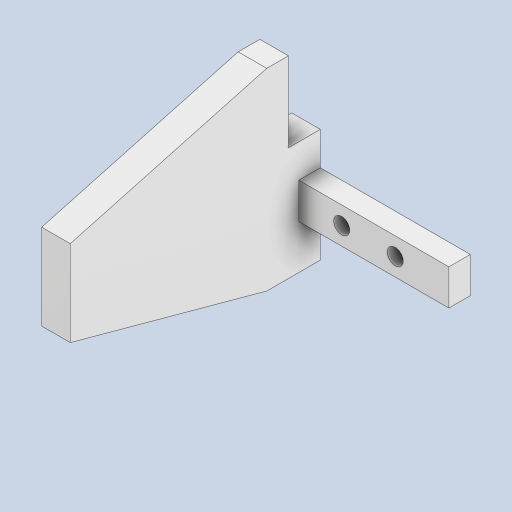
# Autodesk Inventor part: right-nail
Saved by Autodesk Inventor 2023 (Build 270158000, 158)
## iProperties
Created: 2024-11-28
Part Number: right-nail
Material: ABS プラスチック
Document SubType Name: Modeling
Designer: kiyo
Density: 1.06 g/cm^3
Appearance: 滑らか - 白
Author: kiyo
Autodesk Inventor part; units mm, degrees
ref_plane "YZ Plane" through (0, 0, 0) normal (1, 0, 0) x (0, 1, 0)
ref_plane "XZ Plane" through (0, 0, 0) normal (0, 1, 0) x (-1, 0, 0)
ref_plane "XY Plane" through (0, 0, 0) normal (0, 0, 1) x (1, 0, 0)
sketch "スケッチ2" plane through (0, 0, 0) normal (1, 0, 0) x (0, 1, 0)
  line L0 (-50, 41.625) -> (0, 41.625)
  line L1 (0, 41.625) -> (0, 31.625)
  line L2 (0, 31.625) -> (-50, 31.625)
  line L3 (-50, 31.625) -> (-50, 41.625)
  line L4 (0, 31.625) -> (-8, 31.625)
  line L5 (-8, 31.625) -> (-8, 0)
  line L6 (-8, 0) -> (0, 0)
  line L7 (0, 0) -> (0, 31.625)
  circle A0 centre (-20, 36.625) radius 2.25
  circle A1 centre (-35, 36.625) radius 2.25
  line L8 (-8, 31.625) -> (0, 31.625)
  line L9 (0, 31.625) -> (0, 54)
  line L10 (0, 54) -> (-8, 54)
  line L11 (-8, 54) -> (-8, 31.625)
  point P0 (-8, 31.625)
  point P1 (-8, 41.625)
  point P2 (0, 41.625)
  dimension "d7" = 50
  dimension "d8" = 10
  dimension "d10" = 8
  dimension "d11" = 4.5
  dimension "d12" = 4.5
  dimension "d13" = 15
  dimension "d14" = 20
  dimension "d15" = 5
  dimension "d16" = 5
  dimension "d27" = 54
  dimension "d28" = 12.375
  constraints: 24 end point, 6 parallel, 3 horizontal, 3 perpendicular, 2 centre point, 1 coincident, 1 collinear
  measures "d7" distance of L0.start L0.end
  measures "d8" distance between parallel lines of L2 L0
  measures "d10" distance of L5.end L6.end
  measures "d11" diameter of A0
  measures "d12" diameter of A1
  measures "d13" distance of A0.centre A1.centre
  measures "d14" distance from line of L1 A0.centre
  measures "d15" distance from line of L0 A0.centre
  measures "d16" distance from line of L0 A1.centre
  measures "d27" distance between parallel lines of L6 L10
  measures "d28" distance between parallel lines of L0 L10
extrude "押し出し2" add sketch "スケッチ2" along normal blind 6 contours L0 L11 L2 L3
extrude "押し出し5" add sketch "スケッチ2" along normal blind 70 contours L11 L10 L9 L0 | L0 L1 L2 L11 | L2 L7 L6 L5
sketch "スケッチ4" plane through (0, 0, 54) normal (0, 1, 0) x (1, 0, 0)
  line L0 (70, 54) -> (70, 0) projected
  line L1 (70, 15) -> (15, 0)
  line L2 (15, 0) -> (15, 54)
  line L3 (15, 54) -> (70, 39)
  line L4 (0, 54) -> (70, 54) projected
  line L5 (0, 0) -> (70, 0) projected
  line L6 (0, 54) -> (0, 0) projected
  line L7 (0, 22.375) -> (0, 54) projected
  line L8 (0, 54) -> (8.9192, 54)
  line L9 (8.9192, 54) -> (8.9192, 31.7036)
  line L10 (8.9192, 31.7036) -> (0, 31.7036)
  line L11 (0, 31.7036) -> (0, 54)
  dimension "d31" = 15
  dimension "d32" = 15
  dimension "d33" = 15
  constraints: 14 end point, 4 point on line, 3 parallel, 1 horizontal, 1 perpendicular
  measures "d31" distance from line of L5 L1.start
  measures "d32" distance from line of L4 L3.end
  measures "d33" distance between parallel lines of L6 L2
extrude "押し出し6" cut sketch "スケッチ4" against normal blind 8 contours L0 L3 L4 | L0 L5 L1 | L9 L10 L6 L4
sketch "スケッチ5" plane through (0, -8, 41.625) normal (0, -1, 0) x (1, 0, 0)
  line L0 (70, -2.625) -> (70, -26.625) projected
  line L1 (15, -41.625) -> (70, -26.625) projected
  line L2 (70, -2.625) -> (15, 12.375) projected
  line L3 (70, -26.625) -> (15, -41.625) projected
  line L4 (70.01, -26.6223) -> (70.01, -2.6277)
  line L5 (70.01, -26.6223) -> (70, -26.625)
  line L6 (70.01, -2.6277) -> (70, -2.625)
  point P0 (0, -41.625)
  dimension "d36" = 0.01
  constraints: 6 end point, 2 point on line, 1 collinear, 1 vertical
  measures "d36" distance between parallel lines of L4 L0
extrude "押し出し7" add sketch "スケッチ5" against normal blind 8
equation "\"d32\" = d31"
equation "\"d33\" = d31"
